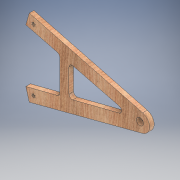
# Autodesk Inventor part: aFrameBase
Saved by Autodesk Inventor 2018 (Build 220112000, 112)
## iProperties
Created: 2017-04-28
Part Number: aFrameBase
Material: Generic
Document SubType Name: Modeling
Designer: admin
Density: 1 g/cm^3
Appearance: Birch - Natural Polished
Author: admin
Autodesk Inventor part; units mm, degrees
ref_plane "YZ Plane" through (0, 0, 0) normal (1, 0, 0) x (0, 1, 0)
ref_plane "XZ Plane" through (0, 0, 0) normal (0, 1, 0) x (-1, 0, 0)
ref_plane "XY Plane" through (0, 0, 0) normal (0, 0, 1) x (1, 0, 0)
ref_plane "Work Plane1" through (0, 0, 0) normal (0, 0, 1) x (1, 0, 0)
sketch "Sketch1" plane through (0, 0, 0) normal (0, 0, 1) x (1, 0, 0)
  line L0 (73.4542, 120.707) -> (75.2544, 119.6677) projected
  arc A0 (73.4542, 120.707) -> (70.7046, 122.2945) centre (72.0794, 121.5007) ccw projected
  line L1 (68.9044, 123.3338) -> (70.7046, 122.2945) projected
  line L2 (68.9044, 125.4125) -> (68.9044, 123.3338) projected
  arc A1 (68.9044, 125.4125) -> (68.9044, 128.5875) centre (68.9044, 127) ccw projected
  line L3 (68.9044, 130.6662) -> (68.9044, 128.5875) projected
  line L4 (70.7046, 131.7055) -> (68.9044, 130.6662) projected
  arc A2 (70.7046, 131.7055) -> (73.4542, 133.293) centre (72.0794, 132.4993) ccw projected
  line L5 (75.2544, 134.3323) -> (73.4542, 133.293) projected
  line L6 (77.0546, 133.293) -> (75.2544, 134.3323) projected
  arc A3 (77.0546, 133.293) -> (79.8042, 131.7055) centre (78.4294, 132.4993) ccw projected
  line L7 (81.6044, 130.6662) -> (79.8042, 131.7055) projected
  line L8 (81.6044, 128.5875) -> (81.6044, 130.6662) projected
  arc A4 (81.6044, 128.5875) -> (81.6044, 125.4125) centre (81.6044, 127) ccw projected
  line L9 (81.6044, 123.3338) -> (81.6044, 125.4125) projected
  line L10 (79.8042, 122.2945) -> (81.6044, 123.3338) projected
  arc A5 (79.8042, 122.2945) -> (77.0546, 120.707) centre (78.4294, 121.5007) ccw projected
  line L11 (75.2544, 119.6677) -> (77.0546, 120.707) projected
  circle A6 centre (75.2544, 127) radius 2.9337 projected
  line L12 (73.4542, -133.293) -> (75.2544, -134.3323) projected
  arc A7 (73.4542, -133.293) -> (70.7046, -131.7055) centre (72.0794, -132.4993) ccw projected
  line L13 (68.9044, -130.6662) -> (70.7046, -131.7055) projected
  line L14 (68.9044, -128.5875) -> (68.9044, -130.6662) projected
  arc A8 (68.9044, -128.5875) -> (68.9044, -125.4125) centre (68.9044, -127) ccw projected
  line L15 (68.9044, -123.3338) -> (68.9044, -125.4125) projected
  line L16 (70.7046, -122.2945) -> (68.9044, -123.3338) projected
  arc A9 (70.7046, -122.2945) -> (73.4542, -120.707) centre (72.0794, -121.5007) ccw projected
  line L17 (75.2544, -119.6677) -> (73.4542, -120.707) projected
  line L18 (77.0546, -120.707) -> (75.2544, -119.6677) projected
  arc A10 (77.0546, -120.707) -> (79.8042, -122.2945) centre (78.4294, -121.5007) ccw projected
  line L19 (81.6044, -123.3338) -> (79.8042, -122.2945) projected
  line L20 (81.6044, -125.4125) -> (81.6044, -123.3338) projected
  arc A11 (81.6044, -125.4125) -> (81.6044, -128.5875) centre (81.6044, -127) ccw projected
  line L21 (81.6044, -130.6662) -> (81.6044, -128.5875) projected
  line L22 (79.8042, -131.7055) -> (81.6044, -130.6662) projected
  arc A12 (79.8042, -131.7055) -> (77.0546, -133.293) centre (78.4294, -132.4993) ccw projected
  line L23 (75.2544, -134.3323) -> (77.0546, -133.293) projected
  circle A13 centre (75.2544, -127) radius 2.9337 projected
  line L24 (75.2544, -127) -> (513.2774, 0) construction
  line L25 (106.8774, 406.4) -> (106.8774, -406.4) projected
  line L26 (513.2774, 0) -> (75.2544, 127) construction
  line L27 (75.2544, 127) -> (50.8591, 134.0732) construction
  line L28 (50.8591, -134.0732) -> (43.7844, -109.6783)
  line L29 (50.8591, -134.0732) -> (57.9322, -158.4684)
  line L30 (57.9322, -158.4684) -> (523.8871, -36.5929)
  circle A14 centre (513.2774, 0) radius 14.2875
  line L31 (513.2774, 0) -> (523.8871, -36.5929) construction
  line L32 (513.2774, 0) -> (552.1398, 0) construction
  arc A15 (523.8871, -36.5929) -> (552.1398, 0) centre (514.3158, 0) ccw
  line L33 (57.9322, 158.4684) -> (523.8871, 36.5929)
  line L34 (513.2774, 0) -> (523.8871, 36.5929) construction
  arc A16 (552.1398, 0) -> (523.8871, 36.5929) centre (514.3158, 0) ccw
  line L35 (75.2544, -127) -> (50.8591, -134.0732) construction
  arc A17 (523.8871, 36.5929) -> (523.8871, -36.5929) centre (514.3158, 0) ccw construction
  line L36 (43.7844, -109.6783) -> (427.9232, -12.3107)
  line L37 (427.9232, 12.3107) -> (43.7859, 109.6779)
  arc A18 (427.9232, -12.3107) -> (427.9232, 12.3107) centre (424.8028, 0) ccw
  line L38 (106.8774, 0) -> (513.2774, 0)
  line L39 (50.8591, 134.0732) -> (57.9322, 158.4684)
  line L40 (50.8591, 134.0732) -> (43.7859, 109.6779)
  line L41 (-111.6762, 0) -> (670.0573, 0) construction
  point P0 (0, 0)
  point P1 (476.4918, 0)
  dimension "d3" = 25.4
  dimension "d18" = 25.4
  dimension "d19" = 25.4
  dimension "d20" = 28.575
  dimension "d21" = 38.1
  dimension "d22" = 90
  dimension "d24" = 38.1
  dimension "d25" = 25.4
  dimension "d28" = 12.7
  dimension "d37" = 406.4
  dimension "d38" = 25.4
  dimension "d39" = 25.4
  constraints: 32 end point, 9 point on circle, 5 centre point, 4 tangent, 3 perpendicular, 2 coincident, 2 collinear, 2 line through centre, 2 point on line, 1 horizontal, 1 midpoint
  measures "d3" distance of L26.end L27.end
  measures "d18" distance of L28.start L28.end
  measures "d19" distance of L28.start L29.end
  measures "d20" diameter of A14
  measures "d21" distance of L31.start L30.end
  measures "d22" angle of L24 L31
  measures "d24" distance of L31.start L33.end
  measures "d25" distance of L28.start L24.start
  measures "d28" radius of A18
  measures "d37" distance of L38.start L24.end
  measures "d38" distance of L33.start L27.end
  measures "d39" distance of L37.end L27.end
extrude "Extrusion3" add sketch "Sketch1" along normal blind 19.05 contours L33 A16 A15 L30 L25 L36 A18 L37 | L25 L37 L40 L39 L33 | L25 L30 L29 L28 L36
sketch "Sketch2" plane through (0, 0, 0) normal (0, 0, -1) x (-1, 0, 0)
  line L0 (-106.8774, 406.4) -> (-106.8774, -406.4) projected
  line L1 (-43.7844, -109.6783) -> (-427.9232, -12.3107) projected
  line L2 (-427.9232, 12.3107) -> (-43.7859, 109.6779) projected
  line L3 (-427.9232, -12.3107) -> (-43.7844, -109.6783) projected
  line L4 (-183.0774, -74.3717) -> (-183.0774, -64.4892) construction
  line L5 (-221.1774, -64.7145) -> (-221.1774, -48.3938) construction
  arc A0 (-236.9978, -60.7045) -> (-221.1774, -48.3938) centre (-233.8774, -48.3938) ccw
  arc A1 (-183.0774, -64.4892) -> (-173.4978, -76.7999) centre (-170.3774, -64.4892) ccw
  arc A2 (-221.1774, 48.3938) -> (-236.9978, 60.7045) centre (-233.8774, 48.3938) ccw
  line L6 (-43.7859, 109.6779) -> (-427.9232, 12.3107) projected
  arc A3 (-173.4978, 76.7998) -> (-183.0774, 64.4891) centre (-170.3774, 64.4891) ccw
  line L7 (-221.1774, -48.3938) -> (-221.1774, 48.3938)
  line L8 (-183.0774, 64.4891) -> (-183.0774, 74.3717) construction
  line L9 (-183.0774, -64.4892) -> (-183.0774, 64.4891)
  line L10 (-221.1774, 48.3938) -> (-221.1774, 64.7145) construction
  point P0 (0, 0)
  dimension "d29" = 76.2
  dimension "d30" = 38.1
  dimension "d33" = 12.7
  dimension "d34" = 12.7
  dimension "d35" = 12.7
  dimension "d36" = 12.7
  constraints: 16 tangent, 12 end point, 12 parallel, 9 point on line, 8 point on circle, 6 vertical, 4 centre point
  measures "d29" distance between parallel lines of L0 L4
  measures "d30" distance between parallel lines of L4 L5
  measures "d33" radius of A0
  measures "d34" radius of A2
  measures "d35" radius of A3
  measures "d36" radius of A1
extrude "Extrusion4" add sketch "Sketch2" against normal up to surface (19.05 mm away) contours A3 L9 A1 L1 A0 L7 A2 L2
body "Solid3"
